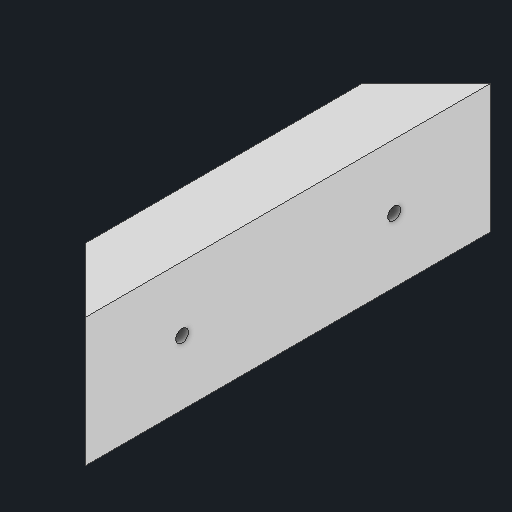
# Autodesk Inventor part: 01_one_side_base_model
Saved by Autodesk Inventor 2024 (Build 280153000, 153)
## iProperties
Created: 2023-05-24
Part Number: 01_one_side_base_model
Material: Generic
Document SubType Name: Modeling
Designer: aasmu
Density: 1 g/cm^3
Appearance: Default
outer_carriage_width: 20.000 mm
outer_carriage_length: 126.000 mm
outer_carriage_height: 40.000 mm
outer_carriage_corner_to_screw: 30.000 mm
outer_carriage_screw_size: 4.000 mm
Author: aasmu
Autodesk Inventor part; units mm, degrees
ref_plane "YZ Plane" through (0, 0, 0) normal (1, 0, 0) x (0, 1, 0)
ref_plane "XZ Plane" through (0, 0, 0) normal (0, 1, 0) x (-1, 0, 0)
ref_plane "XY Plane" through (0, 0, 0) normal (0, 0, 1) x (1, 0, 0)
sketch "Sketch1" plane through (0, 0, 0) normal (0, 1, 0) x (-1, 0, 0)
  line L0 (0.6887, 107.7362) -> (0.6887, -18.2638)
  line L1 (0.6887, -18.2638) -> (20.6887, 1.7362)
  line L2 (20.6887, 1.7362) -> (20.6887, 87.7362)
  line L3 (20.6887, 87.7362) -> (0.6887, 107.7362)
  point P0 (0, 0)
  dimension "d0" = 45
  dimension "d1" = 86
  dimension "d3" = 20
  dimension "d4" = 126
  constraints: 8 end point, 1 parallel, 1 perpendicular, 1 vertical
  measures "d0" angle of L0 L3
  measures "d1" distance of L1.end L2.end
  measures "d3" distance between parallel lines of L0 L2
  measures "d4" distance of L0.start L0.end
extrude "Extrusion1" add sketch "Sketch1" along normal blind 40
sketch "Sketch2" plane through (-20.6887, 0, 1.7362) normal (-1, 0, 0) x (0, 0, 1)
  line L0 (0, 0) -> (0, 40) construction
  line L1 (0, 20) -> (86, 20) construction
  line L2 (86, 0) -> (86, 40) construction
  line L3 (-20, 0) -> (-20, 40) construction
  line L4 (10, 20) -> (-20, 20) construction
  line L5 (76, 20) -> (106, 20) construction
  line L6 (106, 0) -> (106, 40) construction
  line L7 (22, 9.5) -> (28, 9.5)
  line L8 (28, 9.5) -> (28, 30.5)
  line L9 (28, 30.5) -> (22, 30.5)
  line L10 (22, 30.5) -> (22, 9.5)
  line L11 (43, 20) -> (43, 31.7658) construction
  line L12 (64, 9.5) -> (58, 9.5)
  line L13 (58, 9.5) -> (58, 30.5)
  line L14 (58, 30.5) -> (64, 30.5)
  line L15 (64, 30.5) -> (64, 9.5)
  point P0 (-1.7362, 0)
  point P1 (22, 20)
  dimension "d7" = 30
  dimension "d8" = 5
  dimension "d9" = 20
  dimension "d10" = 15
  constraints: 24 end point, 6 midpoint, 4 symmetric about line, 3 point on line, 2 horizontal, 2 parallel, 1 collinear, 1 perpendicular, 1 vertical
  measures "d7" distance of L4.end L4.start
  measures "d10" distance between parallel lines of L11 L8
extrude "Extrusion2" cut sketch "Sketch2" against normal blind 4
hole "Hole1" at (-20.6887, 20, 11.7362) at (-20.6887, 20, 77.7362) direction (1, 0, 0) diameter 4 end through all countersink diameter 7 countersink angle 90
equation "\"d1\" = outer_carriage_innside_length"
equation "\"d3\" = outer_carriage_width"
equation "\"d5\" = outer_carriage_height"
equation "\"d7\" = outer_carriage_corner_to_screw"
equation "\"d8\" = glide_plate_width"
equation "\"d9\" = glide_plate_length"
equation "\"d10\" = outer_carriage_center_to_glideplate"
equation "\"d11\" = glide_plate_height - outer_carriage_to_centerlegg"
equation "\"d13\" = outer_carriage_screw_size"
equation "\"outer_carriage_length\" = d4"
equation "\"outer_carriage_height\" = 40"
equation "\"outer_carriage_width\" = 20"
equation "\"outer_carriage_screw_size\" = 4"
equation "\"outer_carriage_innside_length\" = long_centerlegg_width + 2 * outer_carriage_to_centerlegg"
equation "\"outer_carriage_center_to_glideplate\" = 15"
equation "\"outer_carriage_to_centerlegg\" = 1"
equation "\"outer_carriage_corner_to_screw\" = 30"
equation "\"glide_plate_width\" = 5"
equation "\"glide_plate_length\" = 20"
equation "\"glide_plate_height\" = 5"
equation "\"long_centerlegg_width\" = 84"
body "Solid1"
